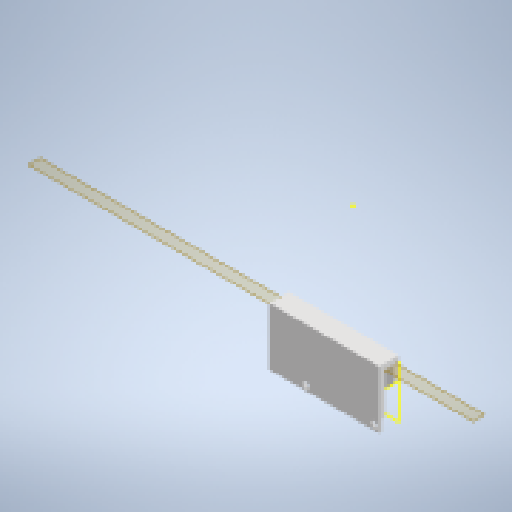
# Autodesk Inventor part: display_holder
Saved by Autodesk Inventor 2024 (Build 280153000, 153)
## iProperties
Created: 2026-03-17
Part Number: display_holder
Material: Generic
Document SubType Name: Modeling
Designer: SEMEN
Density: 1 g/cm^3
Appearance: Default
Author: SEMEN
Autodesk Inventor part; units mm, degrees
ref_plane "YZ Plane" through (0, 0, 0) normal (1, 0, 0) x (0, 1, 0)
ref_plane "XZ Plane" through (0, 0, 0) normal (0, 1, 0) x (-1, 0, 0)
ref_plane "XY Plane" through (0, 0, 0) normal (0, 0, 1) x (1, 0, 0)
ref_plane "Work Plane1" through (149.76, -42.5858, 44.0081) normal (0, 1, 0) x (-1, 0, 0)
sketch "Sketch1" plane through (149.76, -42.5858, 44.0081) normal (0, 1, 0) x (-1, 0, 0)
  line L0 (106, 4) -> (260, 4) projected
  line L1 (106, 0) -> (260, 0) construction
  line L2 (106, 0.5) -> (260, 0.5)
  line L3 (106, 6) -> (260, 6)
  line L4 (106, -1.5) -> (260, -1.5)
  line L5 (174.2008, 6) -> (174.2008, 4)
  line L6 (132.2008, -1.5) -> (132.2008, 0.5)
  line L7 (174.2008, 4) -> (174.2008, 0.5)
  line L8 (174.2008, 0.5) -> (174.2008, -1.5)
  line L9 (132.2008, 4) -> (132.2008, 6)
  line L10 (132.2008, 0.5) -> (132.2008, 4)
  point P0 (149.76, -44.0081)
  dimension "d0" = 0.5
  dimension "d1" = 2
  dimension "d2" = 2
  dimension "d3" = 42
  constraints: 18 end point, 8 point on line, 6 perpendicular, 3 parallel
  measures "d0" distance between parallel lines of L1 L2
  measures "d1" distance between parallel lines of L0 L3
  measures "d2" distance between parallel lines of L2 L4
  measures "d3" distance between parallel lines of L9 L5
extrude "Extrusion1" add sketch "Sketch1" against normal blind 20 contours L9 L3 L5 L0 | L2 L8 L4 L6
sketch "Sketch2" plane through (149.76, -42.5858, 44.0081) normal (0, 1, 0) x (1, 0, 0)
  line L0 (-132.2008, 1.5) -> (-174.2008, 1.5) projected
  line L1 (-174.2008, 1.5) -> (-174.2008, -0.5) projected
  line L2 (-174.2008, -4) -> (-174.2008, -0.5) projected
  line L3 (-174.2008, -4) -> (-174.2008, -6) projected
  line L4 (-174.2008, -6) -> (-132.2008, -6) projected
  line L5 (-132.2008, -6) -> (-132.2008, -4) projected
  line L6 (-132.2008, -0.5) -> (-132.2008, -4) projected
  line L7 (-132.2008, -0.5) -> (-132.2008, 1.5) projected
  point P0 (-149.76, 44.0081)
extrude "Extrusion2" add sketch "Sketch2" along normal blind 2
sketch "Sketch3" plane through (17.5592, -62.5858, 42.5081) normal (0, 0, -1) x (-1, 0, 0)
  line L0 (0, 20) -> (0, 0) projected
  line L1 (0, 2) -> (42, 2) construction
  line L2 (42, 20) -> (42, 0) projected
  line L3 (42, 0) -> (0, 0) projected
  line L4 (28.1005, 0) -> (42, 13.8995)
  point P0 (17.5592, 62.5858)
  point P1 (40, 2)
  point P2 (14, 2)
  dimension "d8" = 2
  dimension "d12" = 7
  dimension "d23" = 45
  dimension "d24" = 2
  dimension "d25" = 26
  constraints: 6 point on line, 4 end point, 1 horizontal
  measures "d8" distance between parallel lines of L3 L1
  measures "d12" distance from line of L4 point (40, 2)
  measures "d23" angle of L2 L4
  measures "d24" distance from line of L2 point (40, 2)
  measures "d25" distance of point (14, 2) point (40, 2)
hole "Hole1" at (3.5592, -60.5858, 42.5081) at (-22.4408, -60.5858, 42.5081) direction (0, 0, 1) diameter 2.4 end through all counterbore diameter 6 counterbore depth 6.35 clearance for "Hex Head Bolt / Nut GOST 12876-67" size "M2" standard "GOST"
sketch "Sketch4" plane through (17.5592, -40.5858, 42.5081) normal (0, 0, -1) x (-1, 0, 0)
  line L0 (0, -2) -> (0, -22) projected
  line L1 (42, -22) -> (0, -22) projected
  line L2 (28.1005, -22) -> (42, -8.1005) projected
  point P0 (17.5592, 40.5858)
  constraints: 2 other
extrude "Extrusion3" cut sketch "Sketch3" against normal up to surface (2 mm away)
body "Solid1"
